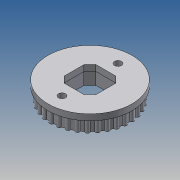
# Autodesk Inventor part: engrane correa dado-motor 2
Saved by Autodesk Inventor 2017 (Build 210142000, 142)
## iProperties
Part Number: engrane correa dado-motor 2
Material: Genérico
Document SubType Name: Modeling
Designer: FABLAB
Density: 1 g/cm^3
Appearance: Blanco
Description: Acrílico corte laser CNC
Author: FABLAB
Autodesk Inventor part; units mm, degrees
ref_plane "YZ Plane" through (0, 0, 0) normal (1, 0, 0) x (0, 1, 0)
ref_plane "XZ Plane" through (0, 0, 0) normal (0, 1, 0) x (-1, 0, 0)
ref_plane "XY Plane" through (0, 0, 0) normal (0, 0, 1) x (1, 0, 0)
sketch "Boceto1" plane through (0, 0, 0) normal (0, 0, 1) x (1, 0, 0)
  line L0 (5, -8) -> (-5, -8) projected
  line L1 (-8, -5) -> (-8, 5) projected
  line L2 (-5, 8) -> (5, 8) projected
  line L3 (8, 5) -> (8, -5) projected
  circle A0 centre (0, 0) radius 19.155
  circle A1 centre (0, 0) radius 16.155 construction
  circle A2 centre (0, 19.155) radius 1
  circle A3 centre (-3.5197, 18.8288) radius 1
  circle A4 centre (-6.9196, 17.8615) radius 1
  circle A5 centre (-10.0838, 16.2859) radius 1
  circle A6 centre (-12.9046, 14.1557) radius 1
  circle A7 centre (-15.286, 11.5435) radius 1
  circle A8 centre (-17.1469, 8.5381) radius 1
  circle A9 centre (-18.4238, 5.242) radius 1
  circle A10 centre (-19.0733, 1.7674) radius 1
  circle A11 centre (-19.0733, -1.7674) radius 1
  circle A12 centre (-18.4238, -5.242) radius 1
  circle A13 centre (-17.1469, -8.5381) radius 1
  circle A14 centre (-15.286, -11.5435) radius 1
  circle A15 centre (-12.9046, -14.1557) radius 1
  circle A16 centre (-10.0838, -16.2859) radius 1
  circle A17 centre (-6.9196, -17.8615) radius 1
  circle A18 centre (-3.5197, -18.8288) radius 1
  circle A19 centre (0, -19.155) radius 1
  circle A20 centre (3.5197, -18.8288) radius 1
  circle A21 centre (6.9196, -17.8615) radius 1
  circle A22 centre (10.0838, -16.2859) radius 1
  circle A23 centre (12.9046, -14.1557) radius 1
  circle A24 centre (15.286, -11.5435) radius 1
  circle A25 centre (17.1469, -8.5381) radius 1
  circle A26 centre (18.4238, -5.242) radius 1
  circle A27 centre (19.0733, -1.7674) radius 1
  circle A28 centre (19.0733, 1.7674) radius 1
  circle A29 centre (18.4238, 5.242) radius 1
  circle A30 centre (17.1469, 8.5381) radius 1
  circle A31 centre (15.286, 11.5435) radius 1
  circle A32 centre (0, 0) radius 21.655 construction
  circle A33 centre (12.9046, 14.1557) radius 1
  circle A34 centre (10.0838, 16.2859) radius 1
  circle A35 centre (6.9196, 17.8615) radius 1
  circle A36 centre (3.5197, 18.8288) radius 1
  line L4 (-5, -8) -> (-8, -5) projected
  line L5 (-8, 5) -> (-5, 8) projected
  line L6 (5, 8) -> (8, 5) projected
  line L7 (8, -5) -> (5, -8) projected
  circle A37 centre (0, 0) radius 21 projected
  circle A38 centre (0, -14) radius 1.7875 projected
  circle A39 centre (0, 14) radius 1.7875 projected
  dimension "d0" = 38.31
  dimension "d4" = 3
  dimension "d16" = 2
  dimension "d19" = 360
  dimension "d24" = 43.31
  dimension "d25" = 3.5348
  dimension "d27" = 2.5
  constraints: 36 centre point, 3 coincident, 2 vertical alignment, 71 other
  measures "d16" diameter of A2
  measures "d24" diameter of A32
  measures "d25" distance of A28.centre A29.centre
extrude "Extrusión1" add sketch "Boceto1" along normal blind 6 contours A0 A27 A26 A25 A24 A23 A22 A21 A20 A19 A18 A17 A16 A15 A14 A13 A12 A11 A10 A9 A8 A7 A6 A5 A4 A3 A2 A36 A35 A34 A33 A31 A30 A29 A28 | A28 A0 | A0 A28 | A27 A0 | A0 A27 | A29 A0 | A0 A29 | A26 A0 | A0 A26 | A30 A0 | A0 A30 | A25 A0 | A0 A25 | A31 A0 | A0 A31 | A24 A0 | A0 A24 | A33 A0 | A0 A33 | A23 A0 | A0 A23 | A34 A0 | A0 A34 | A22 A0 | A0 A22 | A35 A0 | A0 A35 | A21 A0 | A0 A21 | A36 A0 | A0 A36 | A20 A0 | A0 A20 | A2 A0 | A0 A2 | A19 A0 | A0 A19 | A3 A0 | A0 A3 | A18 A0 | A0 A18 | A4 A0 | A0 A4 | A17 A0 | A0 A17 | A5 A0 | A0 A5 | A16 A0 | A0 A16 | A6 A0 | A0 A6 | A15 A0 | A0 A15 | A7 A0 | A0 A7 | A14 A0 | A0 A14 | A8 A0 | A0 A8 | A13 A0 | A0 A13 | A9 A0 | A0 A9 | A12 A0 | A0 A12 | A10 A0 | A0 A10 | A11 A0 | A0 A11
sketch "Boceto3" plane through (0, 0, 6) normal (0, 0, 1) x (1, 0, 0)
  circle A0 centre (0, -14) radius 1.7875 projected
  circle A1 centre (0, 14) radius 1.7875 projected
  line L0 (5, -8) -> (-5, -8) projected
  line L1 (-5, -8) -> (-8, -5) projected
  line L2 (-8, -5) -> (-8, 5) projected
  line L3 (-8, 5) -> (-5, 8) projected
  line L4 (-5, 8) -> (5, 8) projected
  line L5 (5, 8) -> (8, 5) projected
  line L6 (8, 5) -> (8, -5) projected
  line L7 (8, -5) -> (5, -8) projected
  circle A2 centre (0, 0) radius 21 projected
extrude "Extrusión3" add sketch "Boceto3" along normal blind 3 separate body
